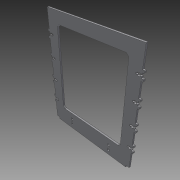
# Autodesk Inventor part: frame_back
Saved by Autodesk Inventor 2014 (Build 180170000, 170)
## iProperties
Created: 2014-03-29
Part Number: frame_back
Material: Plywood, Finish
Document SubType Name: Modeling
Designer: buben
Density: 0.552 g/cm^3
Appearance: Plywood - New
Author: buben
Autodesk Inventor part; units mm, degrees
ref_plane "YZ Plane" through (0, 0, 0) normal (1, 0, 0) x (0, 1, 0)
ref_plane "XZ Plane" through (0, 0, 0) normal (0, 1, 0) x (-1, 0, 0)
ref_plane "XY Plane" through (0, 0, 0) normal (0, 0, 1) x (1, 0, 0)
sketch "Sketch1" plane through (0, 0, 0) normal (0, 1, 0) x (-1, 0, 0)
  line L0 (0, 0) -> (-336, 0)
  line L1 (-336, 0) -> (-336, -404)
  line L2 (-336, -404) -> (0, -404)
  line L3 (0, -404) -> (0, 0)
  line L4 (-48, -40) -> (-288, -40)
  line L5 (-296, -48) -> (-296, -336)
  line L6 (-288, -344) -> (-48, -344)
  line L7 (-40, -336) -> (-40, -48)
  line L8 (-40, -336) -> (-48, -344)
  line L9 (-288, -344) -> (-296, -336)
  line L10 (-296, -48) -> (-288, -40)
  line L11 (-48, -40) -> (-40, -48)
  point P0 (-40, -40)
  point P1 (-296, -40)
  point P2 (-296, -344)
  point P3 (-40, -344)
  dimension "d0" = 404
  dimension "d1" = 336
  dimension "d2" = 8
  dimension "d3" = 8
  dimension "d4" = 8
  dimension "d5" = 8
  dimension "d6" = 8
  dimension "d7" = 8
  dimension "d8" = 8
  dimension "d9" = 8
  dimension "d10" = 40
  dimension "d48" = 40
  dimension "d49" = 40
  dimension "d50" = 60
  constraints: 24 end point, 8 point on line, 4 parallel, 2 perpendicular, 1 horizontal
  measures "d0" distance of L2.end L0.start
  measures "d1" distance of L0.start L0.end
  measures "d2" distance of L7.start point (-40, -344)
  measures "d3" distance of L6.end point (-40, -344)
  measures "d4" distance of L6.start point (-296, -344)
  measures "d5" distance of L5.end point (-296, -344)
  measures "d6" distance of L5.start point (-296, -40)
  measures "d7" distance of L4.end point (-296, -40)
  measures "d8" distance of L4.start point (-40, -40)
  measures "d9" distance of L7.end point (-40, -40)
  measures "d10" distance between parallel lines of L3 L7
  measures "d48" distance between parallel lines of L0 L4
  measures "d49" distance between parallel lines of L1 L5
  measures "d50" distance between parallel lines of L2 L6
extrude "Extrusion1" add sketch "Sketch1" along normal blind 6.5
sketch "Sketch2" plane through (0, 6.5, 0) normal (0, 1, 0) x (1, 0, 0)
  line L0 (0, 0) -> (336, 0) projected
  line L1 (336, 404) -> (0, 404) projected
  line L2 (0, 404) -> (0, 0) projected
  line L3 (16.3, 325.45) -> (16.3, 320.95)
  line L4 (0, 320.95) -> (0, 325.45)
  line L5 (5, 327.95) -> (12.3, 327.95)
  line L6 (12.3, 318.45) -> (5, 318.45)
  line L7 (0, 325.45) -> (5, 325.45)
  line L8 (12.3, 325.45) -> (16.3, 325.45)
  line L9 (16.3, 320.95) -> (12.3, 320.95)
  line L10 (5, 320.95) -> (0, 320.95)
  line L11 (5, 318.45) -> (5, 320.95)
  line L12 (5, 325.45) -> (5, 327.95)
  line L13 (12.3, 327.95) -> (12.3, 325.45)
  line L14 (12.3, 320.95) -> (12.3, 318.45)
  line L15 (16.3, 244.65) -> (16.3, 240.15)
  line L16 (0, 240.15) -> (0, 244.65)
  line L17 (5, 247.15) -> (12.3, 247.15)
  line L18 (12.3, 237.65) -> (5, 237.65)
  line L19 (0, 244.65) -> (5, 244.65)
  line L20 (12.3, 244.65) -> (16.3, 244.65)
  line L21 (16.3, 240.15) -> (12.3, 240.15)
  line L22 (5, 240.15) -> (0, 240.15)
  line L23 (5, 237.65) -> (5, 240.15)
  line L24 (5, 244.65) -> (5, 247.15)
  line L25 (12.3, 247.15) -> (12.3, 244.65)
  line L26 (12.3, 240.15) -> (12.3, 237.65)
  line L27 (16.3, 163.85) -> (16.3, 159.35)
  line L28 (0, 159.35) -> (0, 163.85)
  line L29 (5, 166.35) -> (12.3, 166.35)
  line L30 (12.3, 156.85) -> (5, 156.85)
  line L31 (0, 163.85) -> (5, 163.85)
  line L32 (12.3, 163.85) -> (16.3, 163.85)
  line L33 (16.3, 159.35) -> (12.3, 159.35)
  line L34 (5, 159.35) -> (0, 159.35)
  line L35 (5, 156.85) -> (5, 159.35)
  line L36 (5, 163.85) -> (5, 166.35)
  line L37 (12.3, 166.35) -> (12.3, 163.85)
  line L38 (12.3, 159.35) -> (12.3, 156.85)
  line L39 (16.3, 83.05) -> (16.3, 78.55)
  line L40 (0, 78.55) -> (0, 83.05)
  line L41 (5, 85.55) -> (12.3, 85.55)
  line L42 (12.3, 76.05) -> (5, 76.05)
  line L43 (0, 83.05) -> (5, 83.05)
  line L44 (12.3, 83.05) -> (16.3, 83.05)
  line L45 (16.3, 78.55) -> (12.3, 78.55)
  line L46 (5, 78.55) -> (0, 78.55)
  line L47 (5, 76.05) -> (5, 78.55)
  line L48 (5, 83.05) -> (5, 85.55)
  line L49 (12.3, 85.55) -> (12.3, 83.05)
  line L50 (12.3, 78.55) -> (12.3, 76.05)
  line L51 (168, 404) -> (168, 0) construction
  line L52 (319.7, 325.45) -> (319.7, 320.95)
  line L53 (336, 320.95) -> (336, 325.45)
  line L54 (331, 327.95) -> (323.7, 327.95)
  line L55 (323.7, 318.45) -> (331, 318.45)
  line L56 (336, 325.45) -> (331, 325.45)
  line L57 (323.7, 325.45) -> (319.7, 325.45)
  line L58 (319.7, 320.95) -> (323.7, 320.95)
  line L59 (331, 320.95) -> (336, 320.95)
  line L60 (331, 318.45) -> (331, 320.95)
  line L61 (331, 325.45) -> (331, 327.95)
  line L62 (323.7, 327.95) -> (323.7, 325.45)
  line L63 (323.7, 320.95) -> (323.7, 318.45)
  line L64 (331, 244.65) -> (331, 247.15)
  line L65 (323.7, 237.65) -> (331, 237.65)
  line L66 (319.7, 240.15) -> (323.7, 240.15)
  line L67 (319.7, 244.65) -> (319.7, 240.15)
  line L68 (323.7, 244.65) -> (319.7, 244.65)
  line L69 (331, 237.65) -> (331, 240.15)
  line L70 (331, 247.15) -> (323.7, 247.15)
  line L71 (323.7, 247.15) -> (323.7, 244.65)
  line L72 (323.7, 240.15) -> (323.7, 237.65)
  line L73 (336, 240.15) -> (336, 244.65)
  line L74 (331, 240.15) -> (336, 240.15)
  line L75 (336, 244.65) -> (331, 244.65)
  line L76 (331, 163.85) -> (331, 166.35)
  line L77 (323.7, 156.85) -> (331, 156.85)
  line L78 (319.7, 159.35) -> (323.7, 159.35)
  line L79 (319.7, 163.85) -> (319.7, 159.35)
  line L80 (323.7, 163.85) -> (319.7, 163.85)
  line L81 (331, 156.85) -> (331, 159.35)
  line L82 (331, 166.35) -> (323.7, 166.35)
  line L83 (323.7, 166.35) -> (323.7, 163.85)
  line L84 (323.7, 159.35) -> (323.7, 156.85)
  line L85 (336, 159.35) -> (336, 163.85)
  line L86 (331, 159.35) -> (336, 159.35)
  line L87 (336, 163.85) -> (331, 163.85)
  line L88 (331, 83.05) -> (331, 85.55)
  line L89 (323.7, 76.05) -> (331, 76.05)
  line L90 (319.7, 78.55) -> (323.7, 78.55)
  line L91 (319.7, 83.05) -> (319.7, 78.55)
  line L92 (323.7, 83.05) -> (319.7, 83.05)
  line L93 (331, 76.05) -> (331, 78.55)
  line L94 (331, 85.55) -> (323.7, 85.55)
  line L95 (323.7, 85.55) -> (323.7, 83.05)
  line L96 (323.7, 78.55) -> (323.7, 76.05)
  line L97 (336, 78.55) -> (336, 83.05)
  line L98 (331, 78.55) -> (336, 78.55)
  line L99 (336, 83.05) -> (331, 83.05)
  point P0 (16.3, 323.2)
  point P1 (16.3, 242.4)
  point P2 (16.3, 161.6)
  point P3 (16.3, 80.8)
  point P4 (319.7, 323.2)
  point P5 (319.7, 242.4)
  point P6 (319.7, 161.6)
  point P7 (319.7, 80.8)
  dimension "d13" = 4.5
  dimension "d14" = 2.5
  dimension "d15" = 5
  dimension "d16" = 7.3
  dimension "d17" = 4
  dimension "d18" = 80.8
  dimension "d21" = 80.8
  constraints: 194 end point, 52 symmetric about line, 10 parallel, 6 collinear, 4 perpendicular, 3 horizontal, 3 midpoint, 1 vertical, 75 other
  measures "d13" distance of L3.start L3.end
  measures "d14" distance of L9.end L6.start
  measures "d15" distance of L10.start L4.start
  measures "d16" distance of L6.start L6.end
  measures "d17" distance of L3.end L9.end
  measures "d18" distance from line of L1 point (16.3, 323.2)
  measures "d21" distance of L10.start L23.end
extrude "Extrusion2" cut sketch "Sketch2" against normal through all
sketch "Sketch3" plane through (0, 6.5, 0) normal (0, 1, 0) x (1, 0, 0)
  line L0 (336, 404) -> (0, 404) projected
  line L1 (0, 404) -> (0, 325.45) projected
  line L2 (16.3, 325.45) -> (16.3, 320.95) projected
  line L3 (0, 320.95) -> (0, 244.65) projected
  line L4 (0, 0) -> (336, 0) projected
  line L5 (0, 338.7) -> (-4.5, 338.7)
  line L6 (-6.5, 336.7) -> (-6.5, 332.7)
  line L7 (-4.5, 330.7) -> (0, 330.7)
  line L8 (0, 330.7) -> (0, 338.7)
  line L9 (0, 315.7) -> (-4.5, 315.7)
  line L10 (-6.5, 313.7) -> (-6.5, 309.7)
  line L11 (-4.5, 307.7) -> (0, 307.7)
  line L12 (0, 307.7) -> (0, 315.7)
  arc A0 (-4.5, 338.7) -> (-6.5, 336.7) centre (-4.5, 336.7) ccw
  arc A1 (-6.5, 332.7) -> (-4.5, 330.7) centre (-4.5, 332.7) ccw
  arc A2 (-4.5, 315.7) -> (-6.5, 313.7) centre (-4.5, 313.7) ccw
  arc A3 (-6.5, 309.7) -> (-4.5, 307.7) centre (-4.5, 309.7) ccw
  line L13 (0, 257.9) -> (-4.5, 257.9)
  line L14 (-6.5, 255.9) -> (-6.5, 251.9)
  line L15 (-4.5, 249.9) -> (0, 249.9)
  line L16 (0, 249.9) -> (0, 257.9)
  line L17 (0, 234.9) -> (-4.5, 234.9)
  line L18 (-6.5, 232.9) -> (-6.5, 228.9)
  line L19 (-4.5, 226.9) -> (0, 226.9)
  line L20 (0, 226.9) -> (0, 234.9)
  arc A4 (-4.5, 257.9) -> (-6.5, 255.9) centre (-4.5, 255.9) ccw
  arc A5 (-6.5, 251.9) -> (-4.5, 249.9) centre (-4.5, 251.9) ccw
  arc A6 (-4.5, 234.9) -> (-6.5, 232.9) centre (-4.5, 232.9) ccw
  arc A7 (-6.5, 228.9) -> (-4.5, 226.9) centre (-4.5, 228.9) ccw
  line L21 (0, 177.1) -> (-4.5, 177.1)
  line L22 (-6.5, 175.1) -> (-6.5, 171.1)
  line L23 (-4.5, 169.1) -> (0, 169.1)
  line L24 (0, 169.1) -> (0, 177.1)
  line L25 (0, 154.1) -> (-4.5, 154.1)
  line L26 (-6.5, 152.1) -> (-6.5, 148.1)
  line L27 (-4.5, 146.1) -> (0, 146.1)
  line L28 (0, 146.1) -> (0, 154.1)
  arc A8 (-4.5, 177.1) -> (-6.5, 175.1) centre (-4.5, 175.1) ccw
  arc A9 (-6.5, 171.1) -> (-4.5, 169.1) centre (-4.5, 171.1) ccw
  arc A10 (-4.5, 154.1) -> (-6.5, 152.1) centre (-4.5, 152.1) ccw
  arc A11 (-6.5, 148.1) -> (-4.5, 146.1) centre (-4.5, 148.1) ccw
  line L29 (0, 96.3) -> (-4.5, 96.3)
  line L30 (-6.5, 94.3) -> (-6.5, 90.3)
  line L31 (-4.5, 88.3) -> (0, 88.3)
  line L32 (0, 88.3) -> (0, 96.3)
  line L33 (0, 73.3) -> (-4.5, 73.3)
  line L34 (-6.5, 71.3) -> (-6.5, 67.3)
  line L35 (-4.5, 65.3) -> (0, 65.3)
  line L36 (0, 65.3) -> (0, 73.3)
  arc A12 (-4.5, 96.3) -> (-6.5, 94.3) centre (-4.5, 94.3) ccw
  arc A13 (-6.5, 90.3) -> (-4.5, 88.3) centre (-4.5, 90.3) ccw
  arc A14 (-4.5, 73.3) -> (-6.5, 71.3) centre (-4.5, 71.3) ccw
  arc A15 (-6.5, 67.3) -> (-4.5, 65.3) centre (-4.5, 67.3) ccw
  line L37 (168, 404) -> (168, 0) construction
  line L38 (336, 338.7) -> (340.5, 338.7)
  line L39 (342.5, 336.7) -> (342.5, 332.7)
  line L40 (340.5, 330.7) -> (336, 330.7)
  line L41 (336, 330.7) -> (336, 338.7)
  line L42 (336, 315.7) -> (340.5, 315.7)
  line L43 (342.5, 313.7) -> (342.5, 309.7)
  line L44 (340.5, 307.7) -> (336, 307.7)
  line L45 (336, 307.7) -> (336, 315.7)
  arc A16 (342.5, 336.7) -> (340.5, 338.7) centre (340.5, 336.7) ccw
  arc A17 (340.5, 330.7) -> (342.5, 332.7) centre (340.5, 332.7) ccw
  arc A18 (342.5, 313.7) -> (340.5, 315.7) centre (340.5, 313.7) ccw
  arc A19 (340.5, 307.7) -> (342.5, 309.7) centre (340.5, 309.7) ccw
  line L46 (336, 249.9) -> (336, 257.9)
  line L47 (336, 257.9) -> (340.5, 257.9)
  line L48 (340.5, 249.9) -> (336, 249.9)
  arc A20 (342.5, 255.9) -> (340.5, 257.9) centre (340.5, 255.9) ccw
  line L49 (342.5, 255.9) -> (342.5, 251.9)
  arc A21 (340.5, 249.9) -> (342.5, 251.9) centre (340.5, 251.9) ccw
  line L50 (336, 226.9) -> (336, 234.9)
  line L51 (336, 234.9) -> (340.5, 234.9)
  line L52 (340.5, 226.9) -> (336, 226.9)
  arc A22 (340.5, 226.9) -> (342.5, 228.9) centre (340.5, 228.9) ccw
  line L53 (342.5, 232.9) -> (342.5, 228.9)
  arc A23 (342.5, 232.9) -> (340.5, 234.9) centre (340.5, 232.9) ccw
  line L54 (336, 169.1) -> (336, 177.1)
  line L55 (336, 177.1) -> (340.5, 177.1)
  line L56 (340.5, 169.1) -> (336, 169.1)
  arc A24 (342.5, 175.1) -> (340.5, 177.1) centre (340.5, 175.1) ccw
  line L57 (342.5, 175.1) -> (342.5, 171.1)
  arc A25 (340.5, 169.1) -> (342.5, 171.1) centre (340.5, 171.1) ccw
  line L58 (336, 146.1) -> (336, 154.1)
  line L59 (336, 154.1) -> (340.5, 154.1)
  line L60 (340.5, 146.1) -> (336, 146.1)
  arc A26 (340.5, 146.1) -> (342.5, 148.1) centre (340.5, 148.1) ccw
  line L61 (342.5, 152.1) -> (342.5, 148.1)
  arc A27 (342.5, 152.1) -> (340.5, 154.1) centre (340.5, 152.1) ccw
  line L62 (336, 88.3) -> (336, 96.3)
  line L63 (336, 96.3) -> (340.5, 96.3)
  line L64 (340.5, 88.3) -> (336, 88.3)
  arc A28 (342.5, 94.3) -> (340.5, 96.3) centre (340.5, 94.3) ccw
  line L65 (342.5, 94.3) -> (342.5, 90.3)
  arc A29 (340.5, 88.3) -> (342.5, 90.3) centre (340.5, 90.3) ccw
  line L66 (336, 65.3) -> (336, 73.3)
  line L67 (336, 73.3) -> (340.5, 73.3)
  line L68 (340.5, 65.3) -> (336, 65.3)
  arc A30 (340.5, 65.3) -> (342.5, 67.3) centre (340.5, 67.3) ccw
  line L69 (342.5, 71.3) -> (342.5, 67.3)
  arc A31 (342.5, 71.3) -> (340.5, 73.3) centre (340.5, 71.3) ccw
  point P0 (16.3, 323.2)
  dimension "d28" = 2
  dimension "d29" = 8
  dimension "d30" = 8
  dimension "d31" = 6.5
  dimension "d32" = 15
  dimension "d33" = 7.5
  dimension "d36" = 80.8
  constraints: 130 end point, 64 point on circle, 64 symmetric about line, 32 centre point, 8 tangent, 4 parallel, 3 equal radius, 3 midpoint, 2 horizontal, 2 perpendicular, 2 point on line, 1 collinear, 1 vertical, 100 other
  measures "d28" radius of A0
  measures "d29" distance between parallel lines of L5 L7
  measures "d30" distance between parallel lines of L11 L9
  measures "d31" distance between parallel lines of L1 L6
  measures "d32" distance between parallel lines of L9 L7
  measures "d33" distance from line of point (16.3, 323.2) L7
  measures "d36" distance of L7.end L16.start
extrude "Extrusion3" add sketch "Sketch3" against normal blind 6.5
sketch "Sketch4" plane through (0, 6.5, 0) normal (0, 1, 0) x (1, 0, 0)
  line L0 (336, 338.7) -> (336, 404) projected
  line L1 (336, 404) -> (0, 404) projected
  line L2 (0, 404) -> (0, 338.7) projected
  line L3 (12, 404) -> (324, 404)
  line L4 (324, 404) -> (324, 412)
  line L5 (324, 412) -> (12, 412)
  line L6 (12, 412) -> (12, 404)
  dimension "d43" = 8
  dimension "d44" = 12
  dimension "d45" = 12
  constraints: 8 end point, 2 parallel, 1 horizontal, 1 perpendicular, 1 point on line
  measures "d43" distance of L5.end L3.start
  measures "d44" distance between parallel lines of L2 L6
  measures "d45" distance between parallel lines of L0 L4
extrude "Extrusion4" add sketch "Sketch4" against normal blind 6.5
sketch "Sketch5" plane through (0, 6.5, 0) normal (0, 1, 0) x (1, 0, 0)
  line L0 (336, 338.7) -> (336, 404) projected
  line L1 (324, 412) -> (12, 412) projected
  line L2 (0, 404) -> (0, 338.7) projected
  line L3 (80, 396.6) -> (86.5, 396.6)
  line L4 (86.5, 396.6) -> (86.5, 388.6)
  line L5 (86.5, 388.6) -> (80, 388.6)
  line L6 (80, 388.6) -> (80, 396.6)
  line L7 (80, 373.6) -> (86.5, 373.6)
  line L8 (86.5, 373.6) -> (86.5, 365.6)
  line L9 (86.5, 365.6) -> (80, 365.6)
  line L10 (80, 365.6) -> (80, 373.6)
  line L11 (80, 388.6) -> (86.5, 373.6) construction
  line L12 (80, 373.6) -> (86.5, 388.6) construction
  circle A0 centre (83.25, 381.1) radius 2.25
  line L13 (249.5, 396.6) -> (256, 396.6)
  line L14 (256, 396.6) -> (256, 388.6)
  line L15 (256, 388.6) -> (249.5, 388.6)
  line L16 (249.5, 388.6) -> (249.5, 396.6)
  line L17 (249.5, 373.6) -> (256, 373.6)
  line L18 (256, 373.6) -> (256, 365.6)
  line L19 (256, 365.6) -> (249.5, 365.6)
  line L20 (249.5, 365.6) -> (249.5, 373.6)
  line L21 (249.5, 388.6) -> (256, 373.6) construction
  line L22 (249.5, 373.6) -> (256, 388.6) construction
  circle A1 centre (252.75, 381.1) radius 2.25
  dimension "d51" = 6.5
  dimension "d52" = 8
  dimension "d53" = 15
  dimension "d54" = 4.5
  dimension "d55" = 6.5
  dimension "d56" = 8
  dimension "d57" = 15
  dimension "d58" = 4.5
  dimension "d59" = 15.4
  dimension "d60" = 80
  dimension "d61" = 80
  constraints: 40 end point, 8 parallel, 7 collinear, 4 horizontal, 4 perpendicular, 2 centre point, 2 midpoint
  measures "d51" distance of L3.start L3.end
  measures "d52" distance of L5.end L3.start
  measures "d53" distance between parallel lines of L7 L5
  measures "d54" diameter of A0
  measures "d55" distance of L13.start L13.end
  measures "d56" distance of L21.start L13.start
  measures "d57" distance between parallel lines of L17 L15
  measures "d58" diameter of A1
  measures "d59" distance between parallel lines of L1 L3
  measures "d60" distance between parallel lines of L2 L6
  measures "d61" distance between parallel lines of L0 L14
extrude "Extrusion5" cut sketch "Sketch5" against normal through all
equation "\"d3\" = d2"
equation "\"d4\" = d2"
equation "\"d5\" = d4"
equation "\"d6\" = d2"
equation "\"d7\" = d6"
equation "\"d8\" = d2"
equation "\"d9\" = d8"
equation "\"d48\" = d10"
equation "\"d49\" = d48"
equation "\"d30\" = d29"
equation "\"d33\" = 0.5 * d32"
equation "\"d45\" = d44"
equation "\"d61\" = d60"
body "Solid1"
